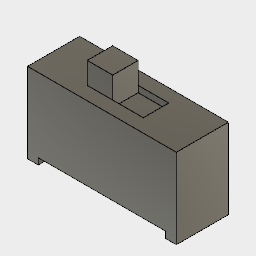
Feather Box V2 (Autodesk Fusion 360 archive; units mm, degrees)
design "Slide Switch"
Autodesk Fusion 360 part; units mm, degrees
note: some values were not read from the file. Chosen so that the rebuilt part matches the saved one: which face or edge a step refers to. Set by a fixed rule: which sketch regions a step uses.
sketch "Sketch1" plane through (0, 0, 0) normal (0, 0, 1) x (1, 0, 0)
  line L0 (0, 0) -> (11.7, 0)
  line L1 (11.7, 0) -> (11.7, -4.1)
  line L2 (11.7, -4.1) -> (0, -4.1)
  line L3 (0, -4.1) -> (0, 0)
  line L4 (5.85, 0) -> (5.85, -4.1) construction
  line L5 (0, -2.05) -> (11.7, -2.05) construction
  line L6 (8.05, -3.05) -> (3.65, -3.05)
  line L7 (3.65, -3.05) -> (3.65, -1.05)
  line L8 (3.65, -1.05) -> (8.05, -1.05)
  line L9 (8.05, -1.05) -> (8.05, -3.05)
  line L10 (8.05, -3.05) -> (3.65, -1.05) construction
  line L11 (3.65, -3.05) -> (8.05, -1.05) construction
  line L12 (3.65, -1.05) -> (5.65, -1.05)
  line L13 (5.65, -1.05) -> (5.65, -3.05)
  line L14 (5.65, -3.05) -> (3.65, -3.05)
  line L15 (3.65, -3.05) -> (3.65, -1.05)
  point P0 (5.85, -2.05)
  dimension "d1" = 11.7
  dimension "d2" = 4.1
  dimension "d3" = 4.4
  dimension "d4" = 2
  dimension "d5" = 2
  measures "d1" distance of L0.start L0.end
  measures "d2" distance of L0.start L2.end
  measures "d3" distance of L7.end L8.end
  measures "d4" distance of L6.end L7.end
  measures "d5" distance of L7.end L12.end
extrude "Extrude1" add sketch "Sketch1" against normal blind 6.3 contours L0 L1 L2 L3 | L6 L8 L9 L13 | L6 L7 L8 L12 L13 L14 L15
extrude "Extrude2" cut sketch "Sketch1" against normal blind 0.5 contours L6 L8 L9 L13 | L6 L7 L8 L12 L13 L14 L15
extrude "Extrude3" add sketch "Sketch1" along normal blind 1.7 and the other way blind 0.5 contours L6 L7 L8 L12 L13 L14 L15
sketch "Sketch2" plane through (0, 0, -6.3) normal (0, 0, -1) x (1, 0, 0)
  line L0 (11.7, 4.1) -> (0, 4.1)
  line L1 (0, 4.1) -> (0, 0)
  line L2 (0, 0) -> (11.7, 0)
  line L3 (11.7, 0) -> (11.7, 4.1)
  line L4 (5.85, 4.1) -> (5.85, 0) construction
  line L5 (0, 2.05) -> (11.7, 2.05) construction
  line L6 (10.85, 0) -> (0.85, 0)
  line L7 (0.85, 0) -> (0.85, 4.1)
  line L8 (0.85, 4.1) -> (10.85, 4.1)
  line L9 (10.85, 4.1) -> (10.85, 0)
  line L10 (10.85, 0) -> (0.85, 4.1) construction
  line L11 (0.85, 0) -> (10.85, 4.1) construction
  point P0 (5.85, 2.05)
  dimension "d13" = 10
  dimension "d14" = 4.1
  measures "d13" distance of L7.end L8.end
  measures "d14" distance of L6.end L7.end
extrude "Extrude4" cut sketch "Sketch2" against normal blind 0.5 contours L0 L2 L6 L7 L8 L9

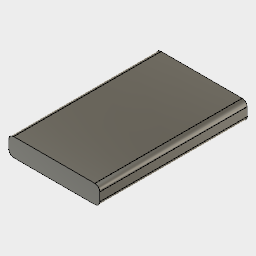
design "2000mAh Battery"
Autodesk Fusion 360 part; units mm, degrees
sketch "Sketch1" plane through (0, 0, 0) normal (0, 0, 1) x (1, 0, 0)
  line L0 (18.5, -30) -> (-18.5, -30)
  line L1 (-18.5, -30) -> (-18.5, 30)
  line L2 (-18.5, 30) -> (18.5, 30)
  line L3 (18.5, 30) -> (18.5, -30)
  line L4 (18.5, -30) -> (-18.5, 30) construction
  line L5 (-18.5, -30) -> (18.5, 30) construction
  dimension "d1" = 60
  dimension "d2" = 37
  measures "d1" distance of L0.end L1.end
  measures "d2" distance of L1.end L2.end
extrude "Extrude1" add sketch "Sketch1" along normal blind 7.5
fillet "Fillet1" radius 2 4 edges at (18.5, 0, 7.5) (18.5, 0, 0) (-18.5, 0, 7.5) (-18.5, 0, 0)

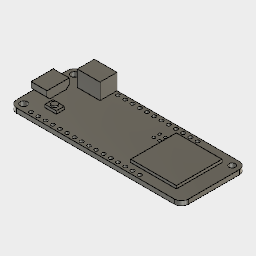
design "Adafruit FONA Feather 32u4"
Autodesk Fusion 360 part; units mm, degrees
sketch "Adafruit Feather 32u4 FONA" plane through (0, 0, 0) normal (0, 0, 1) x (1, 0, 0)
  arc A0 (1.895, 14.93) -> (2.295, 14.58) centre (2.27, 14.955) ccw
  line L0 (0, 8.89) -> (0, 2.54)
  arc A1 (60.325, 20.32) -> (57.785, 22.86) centre (57.785, 20.32) ccw
  arc A2 (2.245, 8.28) -> (1.895, 7.83) centre (2.295, 7.88) ccw
  arc A3 (57.785, 0) -> (60.325, 2.54) centre (57.785, 2.54) ccw
  line L1 (2.845, 14.58) -> (2.295, 14.58)
  line L2 (1.895, 14.93) -> (1.895, 15.13)
  arc A4 (1.895, 7.83) -> (2.245, 7.38) centre (2.295, 7.78) ccw
  arc A5 (0, 2.54) -> (2.54, 0) centre (2.54, 2.54) ccw
  arc A6 (2.845, 14.58) -> (3.195, 14.93) centre (2.845, 14.93) ccw
  arc A7 (2.54, 22.86) -> (0, 20.32) centre (2.54, 20.32) ccw
  line L3 (57.785, 22.86) -> (2.54, 22.86)
  line L4 (60.325, 2.54) -> (60.325, 20.32)
  arc A8 (2.295, 15.48) -> (1.895, 15.13) centre (2.27, 15.105) ccw
  line L5 (3.195, 15.13) -> (3.195, 14.93)
  circle A9 centre (57.785, 20.32) radius 1.1
  line L6 (2.54, 0) -> (57.785, 0)
  arc A10 (3.195, 7.83) -> (2.845, 8.28) centre (2.795, 7.88) ccw
  line L7 (0.508, 13.589) -> (0.508, 9.398)
  line L8 (2.845, 7.38) -> (2.245, 7.38)
  line L9 (0.508, 9.398) -> (0, 8.89)
  line L10 (2.245, 8.28) -> (2.845, 8.28)
  line L11 (0, 20.32) -> (0, 14.097)
  line L12 (0, 14.097) -> (0.508, 13.589)
  arc A11 (2.845, 7.38) -> (3.195, 7.83) centre (2.795, 7.78) ccw
  circle A12 centre (4.445, 13.38) radius 0.35
  arc A13 (3.195, 15.13) -> (2.845, 15.48) centre (2.845, 15.13) ccw
  circle A14 centre (4.445, 9.48) radius 0.35
  line L13 (2.295, 15.48) -> (2.845, 15.48)
  circle A15 centre (35.576, 15.113) radius 0.704
  line L14 (3.795, 9.08) -> (1.295, 9.08)
  circle A16 centre (35.576, 17.145) radius 0.704
  circle A17 centre (39.37, 1.27) radius 0.8382
  line L15 (1.295, 9.08) -> (1.295, 6.58)
  line L16 (1.295, 16.28) -> (1.295, 13.78)
  arc A18 (5.999, 8.13) -> (4.691, 8.13) centre (5.345, 8.13) ccw
  circle A19 centre (35.576, 17.145) radius 0.704
  line L17 (3.795, 16.28) -> (1.295, 16.28)
  line L18 (3.795, 6.58) -> (3.795, 9.08)
  line L19 (1.295, 9.08) -> (1.295, 6.58)
  line L20 (5.999, 6.822) -> (5.999, 8.13)
  line L21 (1.295, 13.78) -> (3.795, 13.78)
  line L22 (4.691, 8.13) -> (4.691, 6.822)
  arc A20 (5.999, 8.13) -> (4.691, 8.13) centre (5.345, 8.13) ccw
  arc A21 (4.691, 6.822) -> (5.999, 6.822) centre (5.345, 6.822) ccw
  line L23 (5.999, 6.822) -> (5.999, 8.13)
  line L24 (3.795, 13.78) -> (3.795, 16.28)
  circle A22 centre (37.576, 17.145) radius 0.704
  line L25 (3.795, 9.08) -> (1.295, 9.08)
  circle A23 centre (37.576, 17.145) radius 0.704
  line L26 (1.295, 13.78) -> (3.795, 13.78)
  arc A24 (4.691, 6.822) -> (5.999, 6.822) centre (5.345, 6.822) ccw
  line L27 (1.295, 16.28) -> (1.295, 13.78)
  line L28 (1.295, 6.58) -> (3.795, 6.58)
  arc A25 (5.999, 16.038) -> (4.691, 16.038) centre (5.345, 16.038) ccw
  line L29 (3.795, 13.78) -> (3.795, 16.28)
  line L30 (5.999, 14.73) -> (5.999, 16.038)
  line L31 (5.999, 14.73) -> (5.999, 16.038)
  arc A26 (4.691, 14.73) -> (5.999, 14.73) centre (5.345, 14.73) ccw
  arc A27 (5.999, 16.038) -> (4.691, 16.038) centre (5.345, 16.038) ccw
  line L32 (4.691, 16.038) -> (4.691, 14.73)
  line L33 (4.691, 8.13) -> (4.691, 6.822)
  line L34 (3.795, 6.58) -> (3.795, 9.08)
  arc A28 (4.691, 14.73) -> (5.999, 14.73) centre (5.345, 14.73) ccw
  line L35 (1.295, 6.58) -> (3.795, 6.58)
  line L36 (4.691, 16.038) -> (4.691, 14.73)
  circle A29 centre (37.576, 15.113) radius 0.704
  circle A30 centre (37.576, 15.113) radius 0.704
  circle A31 centre (35.576, 15.113) radius 0.704
  line L37 (3.795, 16.28) -> (1.295, 16.28)
  circle A32 centre (21.59, 21.59) radius 0.8382
  circle A33 centre (41.91, 1.27) radius 0.8382
  circle A34 centre (44.45, 1.27) radius 0.8382
  circle A35 centre (41.91, 1.27) radius 0.8382
  circle A36 centre (2.54, 20.32) radius 1.758
  circle A37 centre (2.54, 2.54) radius 1.758
  circle A38 centre (2.54, 2.54) radius 1.758
  circle A39 centre (2.54, 20.32) radius 1.758
  circle A40 centre (24.13, 21.59) radius 0.8382
  circle A41 centre (21.59, 21.59) radius 0.8382
  circle A42 centre (24.13, 21.59) radius 0.8382
  circle A43 centre (41.91, 21.59) radius 0.8382
  circle A44 centre (41.91, 21.59) radius 0.8382
  circle A45 centre (44.45, 21.59) radius 0.8382
  circle A46 centre (44.45, 21.59) radius 0.8382
  circle A47 centre (36.83, 21.59) radius 0.8382
  circle A48 centre (19.05, 21.59) radius 0.8382
  circle A49 centre (16.51, 21.59) radius 0.8382
  circle A50 centre (21.59, 1.27) radius 0.8382
  circle A51 centre (21.59, 1.27) radius 0.8382
  circle A52 centre (24.13, 1.27) radius 0.8382
  circle A53 centre (11.43, 1.27) radius 0.8382
  circle A54 centre (19.05, 21.59) radius 0.8382
  circle A55 centre (24.13, 1.27) radius 0.8382
  circle A56 centre (26.67, 1.27) radius 0.8382
  circle A57 centre (16.51, 1.27) radius 0.8382
  circle A58 centre (16.51, 1.27) radius 0.8382
  circle A59 centre (16.51, 21.59) radius 0.8382
  circle A60 centre (39.37, 21.59) radius 0.8382
  circle A61 centre (36.83, 21.59) radius 0.8382
  circle A62 centre (39.37, 21.59) radius 0.8382
  circle A63 centre (31.75, 1.27) radius 0.8382
  circle A64 centre (31.75, 1.27) radius 0.8382
  circle A65 centre (29.21, 1.27) radius 0.8382
  circle A66 centre (29.21, 1.27) radius 0.8382
  circle A67 centre (26.67, 1.27) radius 0.8382
  circle A68 centre (8.89, 1.27) radius 0.8382
  circle A69 centre (34.29, 1.27) radius 0.8382
  circle A70 centre (6.35, 1.27) radius 0.8382
  circle A71 centre (8.89, 1.27) radius 0.8382
  circle A72 centre (6.35, 1.27) radius 0.8382
  circle A73 centre (31.75, 21.59) radius 0.8382
  circle A74 centre (31.75, 21.59) radius 0.8382
  circle A75 centre (34.29, 21.59) radius 0.8382
  circle A76 centre (34.29, 1.27) radius 0.8382
  circle A77 centre (29.21, 21.59) radius 0.8382
  circle A78 centre (34.29, 21.59) radius 0.8382
  circle A79 centre (26.67, 21.59) radius 0.8382
  circle A80 centre (11.43, 1.27) radius 0.8382
  circle A81 centre (39.37, 1.27) radius 0.8382
  circle A82 centre (13.97, 1.27) radius 0.8382
  circle A83 centre (26.67, 21.59) radius 0.8382
  circle A84 centre (36.83, 1.27) radius 0.8382
  circle A85 centre (44.45, 1.27) radius 0.8382
  circle A86 centre (19.05, 1.27) radius 0.8382
  circle A87 centre (19.05, 1.27) radius 0.8382
  circle A88 centre (13.97, 1.27) radius 0.8382
  circle A89 centre (29.21, 21.59) radius 0.8382
  circle A90 centre (36.83, 1.27) radius 0.8382
  circle A91 centre (2.54, 2.54) radius 1.25
  circle A92 centre (2.54, 20.32) radius 1.25
  dimension "d1" = 2.5
  dimension "d2" = 2.5
  measures "d1" diameter of A91
  measures "d2" diameter of A92
extrude "Extrude1" add sketch "Adafruit Feather 32u4 FONA" against normal blind 1.6 contours A0 L1 L2 A6 A8 L5 A13 L13 | L0 A1 A3 A5 A7 L3 L4 L6 L7 L9 L11 L12 | A2 A4 A10 L8 L10 A11 | A12 | A14 | L14 L15 L18 L19 L25 L28 L34 L35 | L16 L17 L21 L24 L26 L27 L29 L37 | A18 L20 L22 A20 A21 L23 A24 L33 | A25 L30 L31 A26 A27 L32 A28 L36 | A36 A39 | A37 A38 makes body 1
move_face "OffsetFaces1" offset 0.203 32 faces at (44.5542, 2.1017, -1.0667) (42.0142, 2.1017, -1.0667) (39.4742, 2.1017, -1.0667) (36.9342, 2.1017, -1.0667) (34.3942, 2.1017, -1.0667) (32.2048, 1.9741, -1.0667) (30.044, 1.1865, -1.0667) (27.504, 1.1865, -1.0667) (24.964, 1.1865, -1.0667) (22.424, 1.1865, -1.0667) (19.884, 1.1865, -1.0667) (17.344, 1.1865, -1.0667) (14.804, 1.1865, -1.0667) (12.264, 1.1865, -1.0667) (9.724, 1.1865, -1.0667) (7.184, 1.1865, -1.0667) (17.3316, 21.4239, -1.0667) (19.8716, 21.4239, -1.0667) (22.4116, 21.4239, -1.0667) (24.9516, 21.4239, -1.0667) (27.4916, 21.4239, -1.0667) (30.0316, 21.4239, -1.0667) (32.2048, 22.2941, -1.0667) (33.6218, 22.0961, -1.0667) (36.1618, 22.0961, -1.0667) (38.7018, 22.0961, -1.0667) (41.2418, 22.0961, -1.0667) (43.7818, 22.0961, -1.0667) (37.958, 15.7044, -1.0667) (35.958, 15.7044, -1.0667) (35.958, 17.7364, -1.0667) (37.958, 17.7364, -1.0667) on bodies 1
sketch "microUSB" plane through (0, 0, 0) normal (0, 0, 1) x (-1, 0, 0)
  circle A0 centre (-36.83, -21.59) radius 0.6352
  circle A1 centre (-44.45, -21.59) radius 0.6352
  circle A2 centre (-29.21, -1.27) radius 0.6352
  circle A3 centre (-26.67, -1.27) radius 0.6352
  circle A4 centre (-8.89, -1.27) radius 0.6352
  circle A5 centre (-35.576, -17.145) radius 0.501
  circle A6 centre (-36.83, -1.27) radius 0.6352
  circle A7 centre (-29.21, -21.59) radius 0.6352
  circle A8 centre (-13.97, -1.27) radius 0.6352
  circle A9 centre (-19.05, -1.27) radius 0.6352
  circle A10 centre (-44.45, -1.27) radius 0.6352
  circle A11 centre (-26.67, -21.59) radius 0.6352
  circle A12 centre (-39.37, -1.27) radius 0.6352
  circle A13 centre (-39.37, -21.59) radius 0.6352
  circle A14 centre (-41.91, -1.27) radius 0.6352
  circle A15 centre (-6.35, -1.27) radius 0.6352
  circle A16 centre (-16.51, -21.59) radius 0.6352
  circle A17 centre (-16.51, -1.27) radius 0.6352
  circle A18 centre (-19.05, -21.59) radius 0.6352
  circle A19 centre (-31.75, -1.27) radius 0.6352
  circle A20 centre (-21.59, -1.27) radius 0.6352
  circle A21 centre (-11.43, -1.27) radius 0.6352
  circle A22 centre (-37.576, -15.113) radius 0.501
  circle A23 centre (-57.785, -20.32) radius 1.1
  circle A24 centre (-2.54, -20.32) radius 1.25
  circle A25 centre (-2.54, -2.54) radius 1.25
  circle A26 centre (-37.576, -17.145) radius 0.501
  circle A27 centre (-35.576, -15.113) radius 0.501
  circle A28 centre (-31.75, -21.59) radius 0.6352
  circle A29 centre (-24.13, -1.27) radius 0.6352
  circle A30 centre (-34.29, -21.59) radius 0.6352
  circle A31 centre (-41.91, -21.59) radius 0.6352
  circle A32 centre (-21.59, -21.59) radius 0.6352
  circle A33 centre (-34.29, -1.27) radius 0.6352
  circle A34 centre (-24.13, -21.59) radius 0.6352
  line L0 (0, -14.097) -> (-0.508, -13.589)
  line L1 (-0.508, -13.589) -> (-0.508, -9.398)
  line L2 (-0.508, -9.398) -> (0, -8.89)
  line L3 (0, -8.89) -> (0, -2.54)
  arc A35 (0, -2.54) -> (-2.54, 0) centre (-2.54, -2.54) ccw
  line L4 (-2.54, 0) -> (-57.785, 0)
  arc A36 (-57.785, 0) -> (-60.325, -2.54) centre (-57.785, -2.54) ccw
  line L5 (-60.325, -2.54) -> (-60.325, -20.32)
  arc A37 (-60.325, -20.32) -> (-57.785, -22.86) centre (-57.785, -20.32) ccw
  line L6 (-57.785, -22.86) -> (-2.54, -22.86)
  arc A38 (-2.54, -22.86) -> (0, -20.32) centre (-2.54, -20.32) ccw
  line L7 (0, -20.32) -> (0, -14.097)
  line L8 (-0.508, -11.4935) -> (-60.325, -11.43) construction
  line L9 (0, -15.391) -> (-5.6, -15.391)
  line L10 (-5.6, -15.391) -> (-5.6, -7.591)
  line L11 (-5.6, -7.591) -> (0, -7.591)
  line L12 (0, -7.591) -> (0, -15.391)
  line L13 (-5.6, -11.491) -> (0, -11.491) construction
  line L14 (0, -14.097) -> (0, -8.89) construction
  dimension "d9" = 11.369
  dimension "d10" = 7.8
  dimension "d11" = 5.6
  measures "d9" distance of L6 L13
  measures "d10" distance of L9.end L10.end
  measures "d11" distance of L9.start L9.end
extrude "Extrude2" add sketch "microUSB" along normal blind 2.95 separate body contours L0 L1 L2 L3 L7 L9 L10 L11 L12 | L0 L1 L2 L12 makes body 2
chamfer "Chamfer1" distance 1 angle 45 2 edges at (2.8, 7.591, 0) (2.8, 15.391, 0) on bodies 2
sketch "JST 2-pin" plane through (0, 0, 0) normal (0, 0, 1) x (-1, 0, 0)
  circle A0 centre (-36.83, -21.59) radius 0.6352
  circle A1 centre (-44.45, -21.59) radius 0.6352
  circle A2 centre (-29.21, -1.27) radius 0.6352
  circle A3 centre (-26.67, -1.27) radius 0.6352
  circle A4 centre (-8.89, -1.27) radius 0.6352
  circle A5 centre (-35.576, -17.145) radius 0.501
  circle A6 centre (-36.83, -1.27) radius 0.6352
  circle A7 centre (-29.21, -21.59) radius 0.6352
  circle A8 centre (-13.97, -1.27) radius 0.6352
  circle A9 centre (-19.05, -1.27) radius 0.6352
  circle A10 centre (-44.45, -1.27) radius 0.6352
  circle A11 centre (-26.67, -21.59) radius 0.6352
  circle A12 centre (-39.37, -1.27) radius 0.6352
  circle A13 centre (-39.37, -21.59) radius 0.6352
  circle A14 centre (-41.91, -1.27) radius 0.6352
  circle A15 centre (-6.35, -1.27) radius 0.6352
  circle A16 centre (-16.51, -21.59) radius 0.6352
  circle A17 centre (-16.51, -1.27) radius 0.6352
  circle A18 centre (-19.05, -21.59) radius 0.6352
  circle A19 centre (-31.75, -1.27) radius 0.6352
  circle A20 centre (-21.59, -1.27) radius 0.6352
  circle A21 centre (-11.43, -1.27) radius 0.6352
  circle A22 centre (-37.576, -15.113) radius 0.501
  circle A23 centre (-57.785, -20.32) radius 1.1
  circle A24 centre (-2.54, -20.32) radius 1.25
  circle A25 centre (-2.54, -2.54) radius 1.25
  circle A26 centre (-37.576, -17.145) radius 0.501
  circle A27 centre (-35.576, -15.113) radius 0.501
  circle A28 centre (-31.75, -21.59) radius 0.6352
  circle A29 centre (-24.13, -1.27) radius 0.6352
  circle A30 centre (-34.29, -21.59) radius 0.6352
  circle A31 centre (-41.91, -21.59) radius 0.6352
  circle A32 centre (-21.59, -21.59) radius 0.6352
  circle A33 centre (-34.29, -1.27) radius 0.6352
  circle A34 centre (-24.13, -21.59) radius 0.6352
  line L0 (0, -14.097) -> (-0.508, -13.589)
  line L1 (-0.508, -13.589) -> (-0.508, -9.398)
  line L2 (-0.508, -9.398) -> (0, -8.89)
  line L3 (0, -8.89) -> (0, -2.54)
  arc A35 (0, -2.54) -> (-2.54, 0) centre (-2.54, -2.54) ccw
  line L4 (-2.54, 0) -> (-57.785, 0)
  arc A36 (-57.785, 0) -> (-60.325, -2.54) centre (-57.785, -2.54) ccw
  line L5 (-60.325, -2.54) -> (-60.325, -20.32)
  arc A37 (-60.325, -20.32) -> (-57.785, -22.86) centre (-57.785, -20.32) ccw
  line L6 (-57.785, -22.86) -> (-2.54, -22.86)
  arc A38 (-2.54, -22.86) -> (0, -20.32) centre (-2.54, -20.32) ccw
  line L7 (0, -20.32) -> (0, -14.097)
  line L8 (-6.92, -22.86) -> (-14.92, -22.86)
  line L9 (-14.92, -22.86) -> (-14.92, -16.86)
  line L10 (-14.92, -16.86) -> (-6.92, -16.86)
  line L11 (-6.92, -16.86) -> (-6.92, -22.86)
  line L12 (-10.92, -22.86) -> (-10.92, -16.86) construction
  dimension "d15" = 8
  dimension "d16" = 6
  dimension "d17" = 10.92
  measures "d15" distance of L8.start L8.end
  measures "d16" distance of L8.end L9.end
  measures "d17" distance of L7 L12
extrude "Extrude3" add sketch "JST 2-pin" along normal blind 5.6 separate body contours L6 L8 L9 L10 L11 makes body 3
sketch "sim800h" plane through (0, 0, 0) normal (0, 0, 1) x (-1, 0, 0)
  circle A0 centre (-36.83, -21.59) radius 0.6352
  circle A1 centre (-44.45, -21.59) radius 0.6352
  circle A2 centre (-29.21, -1.27) radius 0.6352
  circle A3 centre (-26.67, -1.27) radius 0.6352
  circle A4 centre (-8.89, -1.27) radius 0.6352
  circle A5 centre (-35.576, -17.145) radius 0.501
  circle A6 centre (-36.83, -1.27) radius 0.6352
  circle A7 centre (-29.21, -21.59) radius 0.6352
  circle A8 centre (-13.97, -1.27) radius 0.6352
  circle A9 centre (-19.05, -1.27) radius 0.6352
  circle A10 centre (-44.45, -1.27) radius 0.6352
  circle A11 centre (-26.67, -21.59) radius 0.6352
  circle A12 centre (-39.37, -1.27) radius 0.6352
  circle A13 centre (-39.37, -21.59) radius 0.6352
  circle A14 centre (-41.91, -1.27) radius 0.6352
  circle A15 centre (-6.35, -1.27) radius 0.6352
  circle A16 centre (-16.51, -21.59) radius 0.6352
  circle A17 centre (-16.51, -1.27) radius 0.6352
  circle A18 centre (-19.05, -21.59) radius 0.6352
  circle A19 centre (-31.75, -1.27) radius 0.6352
  circle A20 centre (-21.59, -1.27) radius 0.6352
  circle A21 centre (-11.43, -1.27) radius 0.6352
  circle A22 centre (-37.576, -15.113) radius 0.501
  circle A23 centre (-57.785, -20.32) radius 1.1
  circle A24 centre (-2.54, -20.32) radius 1.25
  circle A25 centre (-2.54, -2.54) radius 1.25
  circle A26 centre (-37.576, -17.145) radius 0.501
  circle A27 centre (-35.576, -15.113) radius 0.501
  circle A28 centre (-31.75, -21.59) radius 0.6352
  circle A29 centre (-24.13, -1.27) radius 0.6352
  circle A30 centre (-34.29, -21.59) radius 0.6352
  circle A31 centre (-41.91, -21.59) radius 0.6352
  circle A32 centre (-21.59, -21.59) radius 0.6352
  circle A33 centre (-34.29, -1.27) radius 0.6352
  circle A34 centre (-24.13, -21.59) radius 0.6352
  line L0 (0, -14.097) -> (-0.508, -13.589)
  line L1 (-0.508, -13.589) -> (-0.508, -9.398)
  line L2 (-0.508, -9.398) -> (0, -8.89)
  line L3 (0, -8.89) -> (0, -2.54)
  arc A35 (0, -2.54) -> (-2.54, 0) centre (-2.54, -2.54) ccw
  line L4 (-2.54, 0) -> (-57.785, 0)
  arc A36 (-57.785, 0) -> (-60.325, -2.54) centre (-57.785, -2.54) ccw
  line L5 (-60.325, -2.54) -> (-60.325, -20.32)
  arc A37 (-60.325, -20.32) -> (-57.785, -22.86) centre (-57.785, -20.32) ccw
  line L6 (-57.785, -22.86) -> (-2.54, -22.86)
  arc A38 (-2.54, -22.86) -> (0, -20.32) centre (-2.54, -20.32) ccw
  line L7 (0, -20.32) -> (0, -14.097)
  line L8 (-55.117, -3.43) -> (-39.117, -3.43)
  line L9 (-39.117, -3.43) -> (-39.117, -19.43)
  line L10 (-39.117, -19.43) -> (-55.117, -19.43)
  line L11 (-55.117, -19.43) -> (-55.117, -3.43)
  line L12 (-55.117, -3.43) -> (-39.117, -19.43) construction
  line L13 (-39.117, -3.43) -> (-55.117, -19.43) construction
  point P0 (-47.117, -11.43)
  dimension "d20" = 16
  dimension "d21" = 16
  dimension "d22" = 11.43
  dimension "d23" = 47.117
  measures "d20" distance of L8.end L9.end
  measures "d21" distance of L9.end L10.end
  measures "d22" distance of L4 P0
  measures "d23" distance of L3 P0
extrude "Extrude4" add sketch "sim800h" along normal blind 1 separate body contours L8 L9 L10 L11 makes body 4
sketch "reset switch" plane through (0, 0, 0) normal (0, 0, 1) x (-1, 0, 0)
  circle A0 centre (-36.83, -21.59) radius 0.6352
  circle A1 centre (-44.45, -21.59) radius 0.6352
  circle A2 centre (-29.21, -1.27) radius 0.6352
  circle A3 centre (-26.67, -1.27) radius 0.6352
  circle A4 centre (-8.89, -1.27) radius 0.6352
  circle A5 centre (-35.576, -17.145) radius 0.501
  circle A6 centre (-36.83, -1.27) radius 0.6352
  circle A7 centre (-29.21, -21.59) radius 0.6352
  circle A8 centre (-13.97, -1.27) radius 0.6352
  circle A9 centre (-19.05, -1.27) radius 0.6352
  circle A10 centre (-44.45, -1.27) radius 0.6352
  circle A11 centre (-26.67, -21.59) radius 0.6352
  circle A12 centre (-39.37, -1.27) radius 0.6352
  circle A13 centre (-39.37, -21.59) radius 0.6352
  circle A14 centre (-41.91, -1.27) radius 0.6352
  circle A15 centre (-6.35, -1.27) radius 0.6352
  circle A16 centre (-16.51, -21.59) radius 0.6352
  circle A17 centre (-16.51, -1.27) radius 0.6352
  circle A18 centre (-19.05, -21.59) radius 0.6352
  circle A19 centre (-31.75, -1.27) radius 0.6352
  circle A20 centre (-21.59, -1.27) radius 0.6352
  circle A21 centre (-11.43, -1.27) radius 0.6352
  circle A22 centre (-37.576, -15.113) radius 0.501
  circle A23 centre (-57.785, -20.32) radius 1.1
  circle A24 centre (-2.54, -20.32) radius 1.25
  circle A25 centre (-2.54, -2.54) radius 1.25
  circle A26 centre (-37.576, -17.145) radius 0.501
  circle A27 centre (-35.576, -15.113) radius 0.501
  circle A28 centre (-31.75, -21.59) radius 0.6352
  circle A29 centre (-24.13, -1.27) radius 0.6352
  circle A30 centre (-34.29, -21.59) radius 0.6352
  circle A31 centre (-41.91, -21.59) radius 0.6352
  circle A32 centre (-21.59, -21.59) radius 0.6352
  circle A33 centre (-34.29, -1.27) radius 0.6352
  circle A34 centre (-24.13, -21.59) radius 0.6352
  line L0 (0, -14.097) -> (-0.508, -13.589)
  line L1 (-0.508, -13.589) -> (-0.508, -9.398)
  line L2 (-0.508, -9.398) -> (0, -8.89)
  line L3 (0, -8.89) -> (0, -2.54)
  arc A35 (0, -2.54) -> (-2.54, 0) centre (-2.54, -2.54) ccw
  line L4 (-2.54, 0) -> (-57.785, 0)
  arc A36 (-57.785, 0) -> (-60.325, -2.54) centre (-57.785, -2.54) ccw
  line L5 (-60.325, -2.54) -> (-60.325, -20.32)
  arc A37 (-60.325, -20.32) -> (-57.785, -22.86) centre (-57.785, -20.32) ccw
  line L6 (-57.785, -22.86) -> (-2.54, -22.86)
  arc A38 (-2.54, -22.86) -> (0, -20.32) centre (-2.54, -20.32) ccw
  line L7 (0, -20.32) -> (0, -14.097)
  line L8 (-11.398, -5.077) -> (-7.398, -5.077)
  line L9 (-7.398, -5.077) -> (-7.398, -7.877)
  line L10 (-7.398, -7.877) -> (-11.398, -7.877)
  line L11 (-11.398, -7.877) -> (-11.398, -5.077)
  line L12 (-11.398, -5.077) -> (-7.398, -7.877) construction
  line L13 (-7.398, -5.077) -> (-11.398, -7.877) construction
  circle A39 centre (-9.398, -6.477) radius 1
  point P0 (-9.398, -6.477)
  dimension "d26" = 4
  dimension "d27" = 2.8
  dimension "d28" = 9.398
  dimension "d29" = 6.477
  dimension "d30" = 2
  measures "d26" distance of L9.end L10.end
  measures "d27" distance of L8.end L9.end
  measures "d28" distance of L3 P0
  measures "d29" distance of L4 P0
  measures "d30" diameter of A39
extrude "Extrude5" add sketch "reset switch" along normal blind 1 separate body contours L8 L9 L10 L11 | A39 makes body 5
extrude "Extrude6" add sketch "reset switch" along normal blind 0.5 from surface at 1 contours A39 bodies 5
equation "d6 = ( 0.406 / 2 ) * 1 mm"
named bodies: "pcb", "microUSB", "jst", "sim800h", "reset switch"

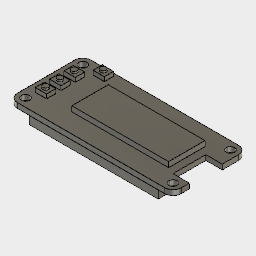
design "Feather OLED Wing"
Autodesk Fusion 360 part; units mm, degrees
sketch "PCB" plane through (0, 0, 0) normal (0, 0, 1) x (1, 0, 0)
  line L0 (0, 0) -> (50.8, 0)
  line L1 (50.8, 0) -> (50.8, 22.86)
  line L2 (50.8, 22.86) -> (0, 22.86)
  line L3 (0, 22.86) -> (0, 0)
  circle A0 centre (2.54, 2.54) radius 1.27
  line L4 (0, 11.43) -> (51, 11.43) construction
  circle A1 centre (2.54, 20.32) radius 1.27
  line L5 (25.4, 22.86) -> (25.4, 0) construction
  circle A2 centre (48.26, 20.32) radius 1.27
  circle A3 centre (48.26, 2.54) radius 1.27
  line L6 (45.72, 15.24) -> (50.8, 15.24)
  line L7 (50.8, 15.24) -> (50.8, 5.08)
  line L8 (50.8, 5.08) -> (45.72, 5.08)
  line L9 (45.72, 5.08) -> (45.72, 15.24)
  dimension "d1" = 50.8
  dimension "d2" = 22.86
  dimension "d3" = 2.54
  dimension "d4" = 2.54
  dimension "d5" = 2.54
  dimension "d9" = 5.08
  dimension "d10" = 10.16
  dimension "d11" = 5.08
  measures "d1" distance of L0.start L0.end
  measures "d2" distance of L0.start L2.end
  measures "d3" diameter of A0
  measures "d4" distance of L0 A0.centre
  measures "d5" distance of L3 A0.centre
  measures "d9" distance of L6.start L6.end
  measures "d10" distance of L6.start L8.end
  measures "d11" distance of L0 L8
extrude "Extrude1" add sketch "PCB" against normal blind 1.6 contours L0 L1 L2 L3 L6 L8 L9 makes body 1
fillet "Fillet1" radius 2.54 4 edges at (0, 22.86, -0.8) (0, 0, -0.8) (50.8, 0, -0.8) (50.8, 22.86, -0.8) on bodies 1
sketch "OLED" plane through (0, 0, 0) normal (0, 0, 1) x (-1, 0, 0)
  circle A0 centre (-2.54, -2.54) radius 1.27
  circle A1 centre (-2.54, -20.32) radius 1.27
  circle A2 centre (-48.26, -2.54) radius 1.27
  circle A3 centre (-48.26, -20.32) radius 1.27
  arc A4 (-50.8, -20.32) -> (-48.26, -22.86) centre (-48.26, -20.32) ccw
  line L0 (-48.26, -22.86) -> (-2.54, -22.86)
  arc A5 (-2.54, -22.86) -> (0, -20.32) centre (-2.54, -20.32) ccw
  line L1 (0, -20.32) -> (0, -2.54)
  arc A6 (0, -2.54) -> (-2.54, 0) centre (-2.54, -2.54) ccw
  line L2 (-2.54, 0) -> (-48.26, 0)
  arc A7 (-48.26, 0) -> (-50.8, -2.54) centre (-48.26, -2.54) ccw
  line L3 (-50.8, -2.54) -> (-50.8, -5.08)
  line L4 (-50.8, -5.08) -> (-45.72, -5.08)
  line L5 (-45.72, -5.08) -> (-45.72, -15.24)
  line L6 (-45.72, -15.24) -> (-50.8, -15.24)
  line L7 (-50.8, -15.24) -> (-50.8, -20.32)
  line L8 (-13.46, -17.27) -> (-43.43, -17.27)
  line L9 (-43.43, -17.27) -> (-43.43, -5.97)
  line L10 (-43.43, -5.97) -> (-13.46, -5.97)
  line L11 (-13.46, -5.97) -> (-13.46, -17.27)
  dimension "d12" = 29.97
  dimension "d13" = 11.3
  dimension "d14" = 5.97
  dimension "d15" = 13.46
  measures "d12" distance of L9.end L10.end
  measures "d13" distance of L8.start L10.end
  measures "d14" distance of L2 L10
  measures "d15" distance of L1 L11
extrude "Extrude2" add sketch "OLED" along normal blind 1.62 separate body contours L8 L9 L10 L11 makes body 2
sketch "buttons" plane through (0, 0, 0) normal (0, 0, 1) x (-1, 0, 0)
  circle A0 centre (-2.54, -2.54) radius 1.27
  circle A1 centre (-2.54, -20.32) radius 1.27
  circle A2 centre (-48.26, -2.54) radius 1.27
  circle A3 centre (-48.26, -20.32) radius 1.27
  arc A4 (-50.8, -20.32) -> (-48.26, -22.86) centre (-48.26, -20.32) ccw
  line L0 (-48.26, -22.86) -> (-2.54, -22.86)
  arc A5 (-2.54, -22.86) -> (0, -20.32) centre (-2.54, -20.32) ccw
  line L1 (0, -20.32) -> (0, -2.54)
  arc A6 (0, -2.54) -> (-2.54, 0) centre (-2.54, -2.54) ccw
  line L2 (-2.54, 0) -> (-48.26, 0)
  arc A7 (-48.26, 0) -> (-50.8, -2.54) centre (-48.26, -2.54) ccw
  line L3 (-50.8, -2.54) -> (-50.8, -5.08)
  line L4 (-50.8, -5.08) -> (-45.72, -5.08)
  line L5 (-45.72, -5.08) -> (-45.72, -15.24)
  line L6 (-45.72, -15.24) -> (-50.8, -15.24)
  line L7 (-50.8, -15.24) -> (-50.8, -20.32)
  line L8 (-6.068, -5.535) -> (-2.568, -5.535)
  line L9 (-2.568, -5.535) -> (-2.568, -8.435)
  line L10 (-2.568, -8.435) -> (-6.068, -8.435)
  line L11 (-6.068, -8.435) -> (-6.068, -5.535)
  line L12 (-6.068, -5.535) -> (-2.568, -8.435) construction
  line L13 (-2.568, -5.535) -> (-6.068, -8.435) construction
  line L14 (-6.068, -9.98) -> (-2.568, -9.98)
  line L15 (-2.568, -9.98) -> (-2.568, -12.88)
  line L16 (-2.568, -12.88) -> (-6.068, -12.88)
  line L17 (-6.068, -12.88) -> (-6.068, -9.98)
  line L18 (-6.068, -9.98) -> (-2.568, -12.88) construction
  line L19 (-2.568, -9.98) -> (-6.068, -12.88) construction
  line L20 (-6.068, -14.425) -> (-2.568, -14.425)
  line L21 (-2.568, -14.425) -> (-2.568, -17.325)
  line L22 (-2.568, -17.325) -> (-6.068, -17.325)
  line L23 (-6.068, -17.325) -> (-6.068, -14.425)
  line L24 (-6.068, -14.425) -> (-2.568, -17.325) construction
  line L25 (-2.568, -14.425) -> (-6.068, -17.325) construction
  line L26 (-10.386, -19.124) -> (-6.886, -19.124)
  line L27 (-6.886, -19.124) -> (-6.886, -22.024)
  line L28 (-6.886, -22.024) -> (-10.386, -22.024)
  line L29 (-10.386, -22.024) -> (-10.386, -19.124)
  line L30 (-10.386, -19.124) -> (-6.886, -22.024) construction
  line L31 (-6.886, -19.124) -> (-10.386, -22.024) construction
  point P0 (-4.318, -6.985)
  point P1 (-4.318, -11.43)
  point P2 (-4.318, -15.875)
  point P3 (-8.636, -20.574)
  dimension "d18" = 3.5
  dimension "d19" = 2.9
  dimension "d20" = 4.318
  dimension "d21" = 6.985
  dimension "d22" = 3.5
  dimension "d23" = 2.9
  dimension "d24" = 4.318
  dimension "d25" = 11.43
  dimension "d26" = 3.5
  dimension "d27" = 2.9
  dimension "d28" = 4.318
  dimension "d29" = 15.875
  dimension "d37" = 3.5
  dimension "d38" = 2.9
  dimension "d39" = 8.636
  dimension "d41" = 20.574
  measures "d18" distance of L9.end L10.end
  measures "d19" distance of L8.end L9.end
  measures "d20" distance of L1 P0
  measures "d21" distance of L2 P0
  measures "d22" distance of L15.end L16.end
  measures "d23" distance of L14.end L15.end
  measures "d24" distance of L1 P1
  measures "d25" distance of L2 P1
  measures "d26" distance of L21.end L22.end
  measures "d27" distance of L20.end L21.end
  measures "d28" distance of L1 P2
  measures "d29" distance of L2 P2
  measures "d37" distance of L27.end L28.end
  measures "d38" distance of L26.end L27.end
  measures "d39" distance of L1 P3
  measures "d41" distance of L2 P3
extrude "Extrude3" add sketch "buttons" along normal blind 1.3 contours L8 L9 L10 L11 | L14 L15 L16 L17 | L20 L21 L22 L23 | L26 L27 L28 L29 bodies 1
sketch "button actuators" plane through (0, 0, 1.3) normal (0, 0, 1) x (-1, 0, 0)
  line L0 (-6.068, -17.325) -> (-2.568, -17.325)
  line L1 (-2.568, -17.325) -> (-2.568, -14.425)
  line L2 (-2.568, -14.425) -> (-6.068, -14.425)
  line L3 (-6.068, -14.425) -> (-6.068, -17.325)
  circle A0 centre (-4.318, -15.875) radius 0.85
  line L4 (-6.068, -12.88) -> (-2.568, -12.88)
  line L5 (-2.568, -12.88) -> (-2.568, -9.98)
  line L6 (-2.568, -9.98) -> (-6.068, -9.98)
  line L7 (-6.068, -9.98) -> (-6.068, -12.88)
  line L8 (-6.068, -8.435) -> (-2.568, -8.435)
  line L9 (-2.568, -8.435) -> (-2.568, -5.535)
  line L10 (-2.568, -5.535) -> (-6.068, -5.535)
  line L11 (-6.068, -5.535) -> (-6.068, -8.435)
  circle A1 centre (-4.318, -11.43) radius 0.85
  circle A2 centre (-4.318, -6.985) radius 0.85
  line L12 (-10.386, -22.024) -> (-6.886, -22.024)
  line L13 (-6.886, -22.024) -> (-6.886, -19.124)
  line L14 (-6.886, -19.124) -> (-10.386, -19.124)
  line L15 (-10.386, -19.124) -> (-10.386, -22.024)
  circle A3 centre (-8.636, -20.574) radius 0.85
  point P0 (-8.636, -20.574)
  dimension "d32" = 1.7
  dimension "d33" = 1.7
  dimension "d34" = 1.7
  dimension "d42" = 1.7
  measures "d32" diameter of A0
  measures "d33" diameter of A1
  measures "d34" diameter of A2
  measures "d42" diameter of A3
extrude "Extrude4" add sketch "button actuators" along normal blind 0.6 contours A0 | A1 | A2 | A3 bodies 1
sketch "header strips" plane through (0, 0, -1.6) normal (0, 0, -1) x (1, 0, 0)
  arc A0 (48.26, -22.86) -> (50.8, -20.32) centre (48.26, -20.32) ccw
  line L0 (50.8, -20.32) -> (50.8, -15.24)
  line L1 (50.8, -15.24) -> (45.72, -15.24)
  line L2 (45.72, -15.24) -> (45.72, -5.08)
  line L3 (45.72, -5.08) -> (50.8, -5.08)
  line L4 (50.8, -5.08) -> (50.8, -2.54)
  arc A1 (50.8, -2.54) -> (48.26, 0) centre (48.26, -2.54) ccw
  line L5 (48.26, 0) -> (2.54, 0)
  arc A2 (2.54, 0) -> (0, -2.54) centre (2.54, -2.54) ccw
  line L6 (0, -2.54) -> (0, -20.32)
  arc A3 (0, -20.32) -> (2.54, -22.86) centre (2.54, -20.32) ccw
  line L7 (2.54, -22.86) -> (48.26, -22.86)
  circle A4 centre (2.54, -2.54) radius 1.27
  circle A5 centre (2.54, -20.32) radius 1.27
  circle A6 centre (48.26, -2.54) radius 1.27
  circle A7 centre (48.26, -20.32) radius 1.27
  line L8 (6.2, 0) -> (46.2, 0)
  line L9 (46.2, 0) -> (46.2, -2.5)
  line L10 (46.2, -2.5) -> (6.2, -2.5)
  line L11 (6.2, -2.5) -> (6.2, 0)
  line L12 (15.2, -22.86) -> (46.2, -22.86)
  line L13 (46.2, -22.86) -> (46.2, -20.36)
  line L14 (46.2, -20.36) -> (15.2, -20.36)
  line L15 (15.2, -20.36) -> (15.2, -22.86)
  dimension "d43" = 40
  dimension "d44" = 2.5
  dimension "d46" = 31
  dimension "d47" = 2.5
  dimension "d51" = 4.6
  dimension "d52" = 4.6
  measures "d43" distance of L8.start L8.end
  measures "d44" distance of L8.start L10.end
  measures "d46" distance of L12.start L12.end
  measures "d47" distance of L12.start L14.end
  measures "d51" distance of L4 L9
  measures "d52" distance of L0 L13
extrude "Extrude5" add sketch "header strips" along normal blind 2.5 separate body contours L7 L12 L13 L14 L15 | L5 L8 L9 L10 L11 makes body 3 at (32.8667, 0, -2.4333) makes body 4 at (35.8667, 22.0267, -1.6)
named bodies: "PCB", "OLED", "header A", "header B"

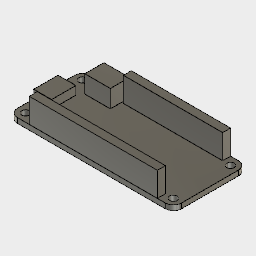
design "Feather BLE with Headers"
Autodesk Fusion 360 part; units mm, degrees
sketch "BLE" plane through (0, 0, 0) normal (0, 0, 1) x (1, 0, 0) in component "Part 1 v1"
  line L0 (51.2, 0) -> (51.2, 22.86)
  line L1 (51.2, 22.86) -> (0, 22.86)
  line L2 (0, 22.86) -> (0, 0)
  line L3 (0, 0) -> (51.2, 0)
  circle A0 centre (48.66, 20.32) radius 1.2
  circle A1 centre (48.66, 2.54) radius 1.2
  circle A2 centre (2.54, 20.32) radius 1.2
  circle A3 centre (2.54, 2.54) radius 1.2
  line L4 (5.6, 7.6) -> (5.6, 15.2)
  line L5 (5.6, 15.2) -> (0, 15.2)
  line L6 (0, 15.2) -> (0, 7.6)
  line L7 (0, 7.6) -> (5.6, 7.6)
  line L8 (5.6, 7.6) -> (0, 15.2) construction
  line L9 (5.6, 15.2) -> (0, 7.6) construction
  line L10 (6.668, 22.86) -> (6.668, 16.86)
  line L11 (6.668, 16.86) -> (14.668, 16.86)
  line L12 (14.668, 16.86) -> (14.668, 22.86)
  line L13 (14.668, 22.86) -> (6.668, 22.86)
  line L14 (6.668, 22.86) -> (14.668, 16.86) construction
  line L15 (6.668, 16.86) -> (14.668, 22.86) construction
  point P0 (25.6, 11.4)
  point P1 (2.8, 11.4)
  point P2 (10.668, 19.86)
  dimension "d11" = 22.86
  dimension "d12" = 51.2
  dimension "d13" = 2.4
  dimension "d14" = 2.54
  dimension "d15" = 2.54
  dimension "d16" = 7.6
  dimension "d17" = 5.6
  dimension "d18" = 6
  dimension "d19" = 8
  dimension "d20" = 10.668
  dimension "d30" = 2.54
  dimension "d31" = 2.54
  dimension "d32" = 2.54
  dimension "d33" = 2.54
  dimension "d34" = 2.54
  dimension "d35" = 2.54
  measures "d11" distance of L1.end L2.end
  measures "d12" distance of L0.end L1.end
  measures "d13" diameter of A0
  measures "d14" distance of L0 A0.centre
  measures "d15" distance of L1 A0.centre
  measures "d16" distance of L5.end L6.end
  measures "d17" distance of L4.end L5.end
  measures "d18" distance of L11.end L12.end
  measures "d19" distance of L10.end L11.end
  measures "d20" distance of L2 P2
  measures "d30" distance of L2 A3.centre
  measures "d31" distance of L3 A3.centre
  measures "d32" distance of L2 A2.centre
  measures "d33" distance of L1 A2.centre
  measures "d34" distance of L3 A1.centre
  measures "d35" distance of L0 A1.centre
extrude "Extrude3" add sketch "BLE" along normal blind 1.6 makes body 1 in component "Part 1 v1"
extrude "Extrude4" add sketch "BLE" along normal blind 7.1 and the other way blind -1.6 separate body contours L1 L10 L11 L12 L13 makes body 2 in component "Part 1 v1"
extrude "Extrude5" add sketch "BLE" along normal blind 4.2 and the other way blind -1.6 separate body contours L2 L4 L5 L6 L7 makes body 3 in component "Part 1 v1"
fillet "Fillet1" radius 2.54 4 edges at (0, 22.86, 0.8) (0, 0, 0.8) (51.2, 0, 0.8) (51.2, 22.86, 0.8) on bodies 1 in component "Part 1 v1"
sketch "headers" plane through (0, 0, 0) normal (0, 0, -1) x (1, 0, 0)
  circle A0 centre (48.66, -2.54) radius 1.2
  circle A1 centre (2.54, -20.32) radius 1.2
  circle A2 centre (2.54, -2.54) radius 1.2
  circle A3 centre (48.66, -20.32) radius 1.2
  arc A4 (48.66, -22.86) -> (51.2, -20.32) centre (48.66, -20.32) ccw
  line L0 (51.2, -20.32) -> (51.2, -2.54)
  arc A5 (51.2, -2.54) -> (48.66, 0) centre (48.66, -2.54) ccw
  line L1 (48.66, 0) -> (2.54, 0)
  arc A6 (2.54, 0) -> (0, -2.54) centre (2.54, -2.54) ccw
  line L2 (0, -2.54) -> (0, -20.32)
  arc A7 (0, -20.32) -> (2.54, -22.86) centre (2.54, -20.32) ccw
  line L3 (2.54, -22.86) -> (48.66, -22.86)
  line L4 (6.2, 0) -> (46.2, 0)
  line L5 (46.2, 0) -> (46.2, -2.5)
  line L6 (46.2, -2.5) -> (6.2, -2.5)
  line L7 (6.2, -2.5) -> (6.2, 0)
  line L8 (46.2, -22.86) -> (15.2, -22.86)
  line L9 (15.2, -22.86) -> (15.2, -20.36)
  line L10 (15.2, -20.36) -> (46.2, -20.36)
  line L11 (46.2, -20.36) -> (46.2, -22.86)
  dimension "d5" = 40
  dimension "d6" = 2.5
  dimension "d8" = 31
  dimension "d9" = 2.5
  dimension "d10" = 5
  dimension "d36" = 5
  measures "d5" distance of L4.start L4.end
  measures "d6" distance of L4.start L6.end
  measures "d8" distance of L8.start L8.end
  measures "d9" distance of L8.start L10.end
  measures "d10" distance of L0 L11
  measures "d36" distance of L0 L5
extrude "Extrude1" add sketch "headers" along normal blind 7.6 separate body contours L3 L8 L9 L10 L11 | L1 L4 L5 L6 L7 makes body 4 at (25.5333, 22.86, -2.5333) makes body 5 at (32.8667, 2.5, -2.5333)
move_body "Move1" bodies 4 5 to x (1, 0, 0) y (0, 1, 0) z (0, 0, 1) at (0, 0, 9.2)
component "Part 1 v1" placed x (1, 0, 0) y (0, 1, 0) z (0, 0, 1) at (0, 0, 0)
equation "d23 = 5.5 mm + 1.6 mm"
named bodies: "feather BLE pcb", "jst", "microUSB", "header 12x", "header 16x"

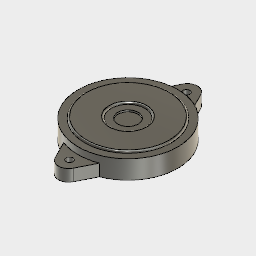
design "Pizero Large"
Autodesk Fusion 360 part; units mm, degrees
sketch "base" plane through (0, 0, 0) normal (0, 0, 1) x (1, 0, 0)
  circle A0 centre (0, 0) radius 14.65
  circle A1 centre (0, 17.2) radius 1
  line L0 (-5.25, 13.677) -> (-2.6683, 18.8354)
  arc A2 (2.6683, 18.8354) -> (-2.6683, 18.8354) centre (0, 17.5) ccw
  line L1 (2.6683, 18.8354) -> (5.25, 13.677)
  line L2 (0, 7.3551) -> (0, 15.8) construction
  line L3 (0, 0) -> (10, 0) construction
  dimension "d1" = 29.3
  dimension "d2" = 2
  dimension "d6" = 10.5
  dimension "d7" = 5.25
  dimension "d20" = 17.2
  measures "d1" diameter of A0
  measures "d2" diameter of A1
  measures "d6" distance of L0.start L1.end
  measures "d7" distance of L1.end L2
  measures "d20" distance of A1.centre L3
extrude "Extrude1" add sketch "base" along normal blind 6 contours A0
extrude "Extrude2" add sketch "base" along normal blind 3.5 contours A0 L0 A2 L1
sketch "top circles" plane through (0, 0, 6) normal (0, 0, 1) x (-1, 0, 0)
  circle A0 centre (0, 0) radius 14.65
  circle A1 centre (0, 0) radius 3
  circle A2 centre (0, 0) radius 5
  circle A3 centre (0, 0) radius 12.65
  dimension "d12" = 6
  dimension "d15" = 2
  dimension "d16" = 2
  measures "d12" diameter of A1
extrude "Extrude3" cut sketch "top circles" against normal blind 1 contours A1
extrude "Extrude4" cut sketch "top circles" against normal blind 0.5
fillet "Fillet1" radius 0.5 2 edges at (4.6616, -1.8081, 6) (11.7939, 4.5744, 6)
mirror "Mirror1" about plane through (0, 0, 0) normal (0, 1, 0) of "Extrude2"
equation "d7 = ( 10.5 / 2 ) * 1 mm"
equation "d20 = ( 34.4 / 2 ) * 1 mm"
